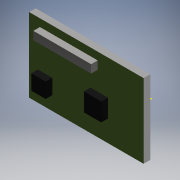
# Autodesk Inventor part: raspberry
Saved by Autodesk Inventor 2019.4 (Build 234330000, 330)
## iProperties
Created: 2020-07-10
Part Number: raspberry
Material: Generic
Document SubType Name: Modeling
Designer: Jorge
Density: 1 g/cm^3
Appearance: Default
Author: Jorge
Autodesk Inventor part; units mm, degrees
ref_plane "YZ Plane" through (0, 0, 0) normal (1, 0, 0) x (0, 1, 0)
ref_plane "XZ Plane" through (0, 0, 0) normal (0, 1, 0) x (-1, 0, 0)
ref_plane "XY Plane" through (0, 0, 0) normal (0, 0, 1) x (1, 0, 0)
sketch "Sketch1" plane through (0, 0, 0) normal (0, 0, 1) x (1, 0, 0)
  line L0 (-5.4839, -45.5191) -> (-92.3615, -45.5191)
  line L1 (-92.3615, -45.5191) -> (-92.3615, 10.7724)
  line L2 (-92.3615, 10.7724) -> (-5.4839, 10.7724)
  line L3 (-5.4839, 10.7724) -> (-5.4839, -45.5191)
  point P0 (0, 0)
  constraints: 8 end point, 2 parallel, 1 horizontal, 1 perpendicular
extrude "Extrusion1" add sketch "Sketch1" along normal blind 5
sketch "Sketch2" plane through (0, 0, 5) normal (0, 0, 1) x (1, 0, 0)
  point P0 (0, 0)
sketch "Sketch3" plane through (0, 0, 5) normal (0, 0, 1) x (1, 0, 0)
  line L0 (-40.3465, 5.0142) -> (-84.1809, 5.0142)
  line L1 (-84.1809, 5.0142) -> (-84.1809, -1.1473)
  line L2 (-84.1809, -1.1473) -> (-40.3465, -1.1473)
  line L3 (-40.3465, -1.1473) -> (-40.3465, 5.0142)
  line L4 (-74.8507, -23.6806) -> (-85.7653, -23.6806)
  line L5 (-85.7653, -23.6806) -> (-85.7653, -35.1234)
  line L6 (-85.7653, -35.1234) -> (-74.8507, -35.1234)
  line L7 (-74.8507, -35.1234) -> (-74.8507, -23.6806)
  line L8 (-32.6006, -15.5827) -> (-45.8038, -15.5827)
  line L9 (-45.8038, -15.5827) -> (-45.8038, -29.402)
  line L10 (-45.8038, -29.402) -> (-32.6006, -29.402)
  line L11 (-32.6006, -29.402) -> (-32.6006, -15.5827)
  point P0 (0, 0)
  constraints: 24 end point, 6 parallel, 3 horizontal, 3 perpendicular
extrude "Extrusion2" add sketch "Sketch3" along normal blind 5
body "Solid1"
